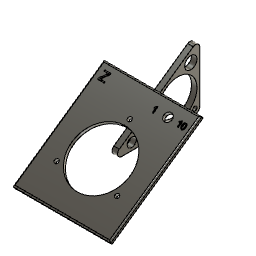
cnc3018_ctrl v33 (Autodesk Fusion 360 design; units mm, degrees)
Autodesk Fusion 360 part; units mm, degrees
ref_plane "WorkPlane2" through (12.125, 0, 0) normal (0, -0.573576, 0.819152) x (1, 0, 0)
sketch "z-plate" plane through (0, 0, 0) normal (0, -0.573576, 0.819152) x (1, 0, 0)
  circle A0 centre (0, 0) radius 21.25
  line L0 (0, 0) -> (0, 36.3774) construction
  circle A1 centre (0, 25.4) radius 1.5
  line L1 (0, 0) -> (-31.5038, -18.1887) construction
  circle A2 centre (-21.997, -12.7) radius 1.5
  line L2 (0, 0) -> (31.5038, -18.1887) construction
  circle A3 centre (21.997, -12.7) radius 1.5
  circle A4 centre (0, 0) radius 30.5 construction
  line L3 (-35.5, 45.5) -> (35.5, 45.5)
  line L4 (35.5, 45.5) -> (35.5, -35.5)
  line L5 (35.5, -35.5) -> (-35.5, -35.5)
  line L6 (-35.5, -35.5) -> (-35.5, 45.5)
  line L7 (12.5, 40.5) -> (25.5, 40.5)
  line L8 (25.5, 40.5) -> (25.5, 32)
  line L9 (25.5, 32) -> (12.5, 32)
  line L10 (12.5, 32) -> (12.5, 40.5)
  line L11 (12.5, 40.5) -> (25.5, 32) construction
  circle A5 centre (19, 36.25) radius 3
  line L12 (6, 36.25) -> (32, 36.25) construction
  line L13 (25.5, 32) -> (32, 32) construction
  line L14 (32, 32) -> (32, 40.5) construction
  line L15 (32, 40.5) -> (25.5, 40.5) construction
  line L16 (25.5, 40.5) -> (25.5, 32) construction
  line L17 (6, 32) -> (12.5, 32) construction
  line L18 (12.5, 32) -> (12.5, 40.5) construction
  line L19 (12.5, 40.5) -> (6, 40.5) construction
  line L20 (6, 40.5) -> (6, 32) construction
  line L21 (-35.5, 30.6686) -> (-21.9667, 30.6686) construction
  line L22 (-21.9667, 30.6686) -> (-21.9667, 45.5) construction
  line L23 (-21.9667, 45.5) -> (-35.5, 45.5) construction
  line L24 (-35.5, 45.5) -> (-35.5, 30.6686) construction
  dimension "d1" = 42.5
  dimension "d4" = 3
  dimension "d5" = 25.4
  dimension "d7" = 360
  dimension "d8" = 61
  dimension "d9" = 5
  dimension "d10" = 5
  dimension "d11" = 5
  dimension "d15" = 13
  dimension "d16" = 8.5
  dimension "d17" = 6
  dimension "d18" = 5
  dimension "d19" = 10
  dimension "d20" = 15
  dimension "d21" = 26
  dimension "d22" = 4
  dimension "d23" = 4
  dimension "d29" = 6
  dimension "enc_panel_h" = 81
  dimension "enc_panel_w" = 71
  text T0 "10" font "Arial" height 4 align right middle in box 6.5 x 8.5 at (25.5, 32) x (1, 0) y (0, 1) spacing 1 kerned
  text T1 "1" font "Arial" height 4 align centre middle in box 6.5 x 8.5 at (6, 32) x (1, 0) y (0, 1) spacing 1 kerned
  text T2 "Z" font "Arial" height 6 align centre middle in box 13.5333 x 14.8314 at (-35.5, 30.6686) x (1, 0) y (0, 1) spacing 1 kerned
  constraint coincident A0.centre L0.start
  constraint vertical L0
  constraint coincident L0 A1.centre
  constraint horizontal L3
  constraint vertical L4
  constraint horizontal L5
  constraint vertical L6
  constraint horizontal L7
  constraint vertical L8
  constraint horizontal L9
  constraint vertical L10
  constraint midpoint L11 A5.centre
  constraint perpendicular L8 L12
  constraint midpoint A5.centre L12
  constraint coincident L7.end
  constraint coincident L7.start
  constraint coincident L3.start
  measures "d1" diameter of A0
  measures "d4" diameter of A1
  measures "d5" distance of A0.centre A1.centre
  measures "d8" diameter of A4
  measures "d9" distance of A4 L6
  measures "d10" distance of A4 L4
  measures "d11" distance of A4 L5
  measures "d15" distance of L7.start L7.end
  measures "d16" distance of L7.start L9.end
  measures "d17" diameter of A5
  measures "d18" distance of L3 L7
  measures "d19" distance of L4 L8
  measures "d20" distance of A4 L3
  measures "d21" distance of L12.start L12.end
  measures "enc_panel_h" distance of L3 L5
  measures "enc_panel_w" distance of L4 L6
extrude "Extrude1" add sketch "z-plate" along normal blind 2.5 contours L3 L4 L5 L6 | L7 L8 L9 L10 makes body 1
extrude "Extrude2" add sketch "z-plate" along normal blind 0.5 from surface at 2.5 text T1 T0 T2 bodies 1
fillet "Fillet3" radius 1 4 edges at (0, 35.8375, 28.1456) (35.5, 2.6618, 4.9158) (0, -30.5138, -18.3141) (-35.5, 2.6618, 4.9158) on bodies 1
sketch "angle plate" plane through (0, 0, 0) normal (1, 0, 0) x (0, 1, 0)
  line L0 (0, 0) -> (66.3513, 0)
  line L1 (66.3513, 0) -> (66.3513, 46.4597)
  line L2 (66.3513, 46.4597) -> (0, 0)
  line L3 (5, 0) -> (5, 3.501)
  line L4 (66.9249, 45.6405) -> (0.5736, -0.8192)
  line L5 (0, 1) -> (66.3513, 1)
  line L6 (4, 0) -> (4, 3.501)
  line L7 (65.3513, 0) -> (65.3513, 46.4597)
  circle A0 centre (50.4458, 15.9055) radius 14.9055
  circle A1 centre (50.4458, 15.9055) radius 13.9055
  line L8 (50.4458, 15.9055) -> (0, 0) construction
  line L9 (36.2302, 11.4233) -> (32.9437, 21.8467) construction
  circle A2 centre (28.5875, 9.0136) radius 8.0136
  circle A3 centre (28.5875, 9.0136) radius 7.0136
  line L10 (20.9448, 6.6039) -> (19.1779, 12.2077) construction
  circle A4 centre (16.8359, 5.3083) radius 4.3083
  circle A5 centre (16.8359, 5.3083) radius 3.3083
  line L11 (66.3513, 46.4597) -> (50.4458, 15.9055) construction
  line L12 (57.3284, 29.1268) -> (49.3055, 33.3033) construction
  circle A6 centre (59.8627, 33.9953) radius 5.4886
  circle A7 centre (59.8627, 33.9953) radius 4.4886
  line L13 (50.4458, 15.9055) -> (66.3513, 0) construction
  line L14 (60.9856, 5.3657) -> (56.6199, 1) construction
  circle A8 centre (62.7939, 3.5574) radius 2.5574
  circle A9 centre (62.7939, 3.5574) radius 1.5574
  dimension "d36" = 35
  dimension "d37" = 81
  dimension "d38" = 5
  dimension "d40" = -1
  dimension "d41" = -1
  dimension "d44" = -1
  dimension "d49" = -1
  dimension "d62" = -1
  dimension "d67" = -1
  dimension "d68" = -1
  dimension "d69" = -1
  dimension "d75" = -1
  constraint coincident L0.start L2.end
  constraint horizontal L0
  constraint perpendicular L0 L1
  constraint coincident L0 L3.start
  constraint coincident L2 L3.end
  constraint perpendicular L0 L3
  constraint tangent L4 A0
  constraint tangent L7 A0
  constraint tangent L5 A0
  constraint coincident A0.centre A1.centre
  constraint coincident A0 L9.start
  constraint coincident L8 L9.start
  constraint coincident L4 L9.end
  constraint tangent A0 L9
  constraint tangent L4 A2
  constraint tangent L5 A2
  constraint tangent L9 A2
  constraint coincident A2 L10.start
  constraint coincident L8 L10.start
  constraint coincident L4 L10.end
  constraint tangent A2 L10
  constraint tangent L4 A4
  constraint tangent L5 A4
  constraint tangent L10 A4
  constraint coincident A0 L12.start
  constraint coincident L11 L12.start
  constraint coincident L4 L12.end
  constraint tangent A0 L12
  constraint tangent L7 A6
  constraint tangent L4 A6
  constraint tangent L12 A6
  constraint coincident A0 L14.start
  constraint coincident L13 L14.start
  constraint coincident L5 L14.end
  constraint tangent A0 L14
  constraint tangent L7 A8
  constraint tangent L5 A8
  constraint tangent L14 A8
  measures "d36" angle of L0 L2
  measures "d37" distance of L1.end L0.start
  measures "d38" distance of L0.start L3.start
extrude "Extrude7" add sketch "angle plate" along normal blind 4 separate body contours L0 L3 L5 L6 | L0 L3 L5 L7 | L3 L4 L5 L6 | L0 L1 L5 L7 | L3 L4 L5 A4 | L2 L3 L4 L6 | L1 L4 L5 L7 | L5 L7 A8 | L2 L3 L4 L7 | L5 A2 A4 | A4 | L5 A0 A8 | A8 | L7 A0 A8 | L4 A2 A4 | L5 A0 A2 | A2 | L1 L2 L4 L7 | A0 | L7 A0 A6 | L4 A0 A2 | L4 L7 A6 | A6 | L4 A0 A6 makes body 2
fillet "Fillet2" radius 3 4 edges at (2, 66.3513, 46.4597) (2, 4, 2.8008) (2, 4, 0) (2, 66.3513, 0) on bodies 2
equation "d1 = enc_hole"
equation "enc_bolt = 3 mm"
equation "enc_hole = 42.5 mm"
equation "d4 = enc_bolt"
equation "d5 = ( 50.8 / 2 ) * 1 mm"
equation "d10 = d9"
equation "d11 = d9"
equation "switch_w = 13 mm"
equation "switch_l = 8.5 mm"
equation "switch_hole = 6 mm"
equation "d15 = switch_w"
equation "d16 = switch_l"
equation "d17 = switch_hole"
equation "d18 = d9"
equation "d19 = d9 * 2"
equation "d21 = 2 * switch_w"
equation "d36 = panel_angle"
equation "d37 = enc_panel_h"
equation "d41 = d40"
equation "d44 = d40"
equation "d49 = d40"
equation "d62 = d40"
equation "d67 = d40"
equation "d68 = d40"
equation "d69 = d40"
equation "panel_angle = 35 deg"
equation "d72 = panel_angle"
equation "d75 = d40"
named bodies: "z-plate", "angle plate"
